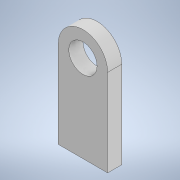
# Autodesk Inventor part: planetenstab
Saved by Autodesk Inventor 2021 (Build 250183000, 183)
## iProperties
Created: 2021-01-26
Part Number: planetenstab
Material: Generisch
Document SubType Name: Modeling
Designer: LETPJG
Density: 1 g/cm^3
Appearance: Vorgabe
Author: LETPJG
Autodesk Inventor part; units mm, degrees
ref_plane "YZ Plane" through (0, 0, 0) normal (1, 0, 0) x (0, 1, 0)
ref_plane "XZ Plane" through (0, 0, 0) normal (0, 1, 0) x (-1, 0, 0)
ref_plane "XY Plane" through (0, 0, 0) normal (0, 0, 1) x (1, 0, 0)
sketch "Skizze1" plane through (0, 0, 0) normal (0, 0, 1) x (1, 0, 0)
  line L0 (3.5, 6.171) -> (3.5, -6.171)
  line L1 (3.5, -6.171) -> (-3.5, -6.171)
  line L2 (-3.5, -6.171) -> (-3.5, 6.171)
  arc A0 (3.5, 6.171) -> (-3.5, 6.171) centre (0, 6.171) ccw
  circle A1 centre (0, 6.171) radius 2
  point P0 (0, 0)
  point P1 (-3.5, 0)
  constraints: 6 end point, 2 centre point, 2 coincident, 2 point on circle, 1 horizontal alignment, 1 midpoint, 1 parallel, 1 vertical alignment
extrude "Extrusion1" add sketch "Skizze1" against normal blind 2
